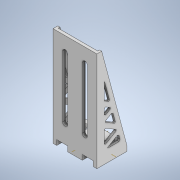
# Autodesk Inventor part: Bottom
Saved by Autodesk Inventor 2020 (Build 240168000, 168)
## iProperties
Created: 2019-08-01
Part Number: Bottom
Material: Generic
Document SubType Name: Modeling
Designer: Alex
Density: 1 g/cm^3
Appearance: Default
Author: Alex
Autodesk Inventor part; units mm, degrees
ref_plane "YZ Plane" through (0, 0, 0) normal (1, 0, 0) x (0, 1, 0)
ref_plane "XZ Plane" through (0, 0, 0) normal (0, 1, 0) x (-1, 0, 0)
ref_plane "XY Plane" through (0, 0, 0) normal (0, 0, 1) x (1, 0, 0)
sketch "Sketch1" plane through (0, 0, 0) normal (0, 1, 0) x (-1, 0, 0)
  line L0 (30, -20) -> (-30, -20)
  line L1 (-30, -20) -> (-30, 20)
  line L2 (-30, 20) -> (30, 20)
  line L3 (30, 20) -> (30, -20)
  line L4 (17.5, -11) -> (17.5, 5) construction
  line L5 (22, -11) -> (22, 5)
  line L6 (13, 5) -> (13, -11)
  arc A0 (13, -11) -> (22, -11) centre (17.5, -11) ccw
  arc A1 (22, 5) -> (13, 5) centre (17.5, 5) ccw
  line L7 (-17.5, -11) -> (-17.5, 5) construction
  line L8 (-13, -11) -> (-13, 5)
  line L9 (-22, 5) -> (-22, -11)
  arc A2 (-22, -11) -> (-13, -11) centre (-17.5, -11) ccw
  arc A3 (-13, 5) -> (-22, 5) centre (-17.5, 5) ccw
  line L10 (0, -28) -> (0, 28) construction
  line L11 (42, 0) -> (-42, 0) construction
  point P0 (0, 0)
  point P1 (17.5, -3)
  point P2 (-17.5, -3)
  dimension "d0" = 60
  dimension "d1" = 40
  dimension "d2" = 4.5
  dimension "d3" = 9
  dimension "d4" = 15
  dimension "d5" = 35
  constraints: 24 end point, 8 point on circle, 8 tangent, 6 parallel, 4 centre point, 2 midpoint, 1 equal radius, 1 horizontal, 1 horizontal alignment, 1 perpendicular, 1 vertical, 3 other
  measures "d0" distance of L1.end L2.end
  measures "d1" distance of L0.end L1.end
  measures "d2" radius of A0
  measures "d3" distance from line of L0 L4.start
  measures "d4" distance from line of L4.end L2
  measures "d5" distance of point (-17.5, -3) point (17.5, -3)
extrude "Extrusion1" add sketch "Sketch1" along normal blind 4
sketch "Sketch2" plane through (0, 4, 0) normal (0, 1, 0) x (1, 0, 0)
  line L0 (-30, -20) -> (30, -20) construction
  line L1 (30, -20) -> (30, 20) construction
  line L2 (30, 20) -> (-30, 20) construction
  line L3 (-30, 20) -> (-30, -20) construction
  line L4 (13, -5) -> (13, 11) construction
  arc A0 (22, 11) -> (13, 11) centre (17.5, 11) ccw construction
  line L5 (22, 11) -> (22, -5) construction
  arc A1 (13, -5) -> (22, -5) centre (17.5, -5) ccw construction
  arc A2 (-22, -5) -> (-13, -5) centre (-17.5, -5) ccw construction
  line L6 (-22, -5) -> (-22, 11) construction
  arc A3 (-13, 11) -> (-22, 11) centre (-17.5, 11) ccw construction
  line L7 (-13, 11) -> (-13, -5) construction
  line L8 (30, -20) -> (30, 20) construction
  line L9 (30, -20) -> (30, 20)
  line L10 (30, 20) -> (-30, 20) construction
  line L11 (27, 20) -> (27, -16)
  line L12 (27, -16) -> (-27, -16)
  line L13 (-27, -16) -> (-27, 20)
  line L14 (-30, 20) -> (-30, -20)
  line L15 (-30, -20) -> (30, -20) projected
  line L16 (-30, -20) -> (30, -20)
  line L17 (30, 20) -> (27, 20)
  line L18 (-27, 20) -> (-30, 20)
  line L19 (0, 38.5) -> (0, -38.5) construction
  point P0 (0, 0)
  dimension "d9" = 4
  dimension "d10" = 3
  constraints: 16 end point, 3 collinear, 3 perpendicular, 2 point on line, 1 vertical, 1 other
  measures "d9" distance between parallel lines of L0 L12
  measures "d10" distance between parallel lines of L11 L1
extrude "Extrusion2" add sketch "Sketch2" along normal blind 125
draft "FaceDraft1" angle 15 pull direction (0, 1, 0) fixed plane through (-4.3333, 4, -0.3333) normal (0, 1, 0) faces at (29, 44.3333, -20)
sketch "Sketch3" plane through (-30, 0, 20) normal (0, 0, 1) x (1, 0, 0)
  line L0 (0, 0) -> (60, 0) construction
  line L1 (60, 0) -> (60, 129) construction
  line L2 (0, 129) -> (60, 129) construction
  line L3 (0, 0) -> (0, 129) construction
  line L4 (16.5, 109) -> (16.5, 25) construction
  line L5 (13, 109) -> (13, 25)
  line L6 (20, 25) -> (20, 109)
  arc A0 (20, 109) -> (13, 109) centre (16.5, 109) ccw
  arc A1 (13, 25) -> (20, 25) centre (16.5, 25) ccw
  line L7 (43.5, 109) -> (43.5, 25) construction
  line L8 (40, 109) -> (40, 25)
  line L9 (47, 25) -> (47, 109)
  arc A2 (47, 109) -> (40, 109) centre (43.5, 109) ccw
  arc A3 (40, 25) -> (47, 25) centre (43.5, 25) ccw
  line L10 (0, 129) -> (60, 129) construction
  line L11 (30, 129) -> (30, 0) construction
  point P0 (16.5, 67)
  point P1 (43.5, 67)
  dimension "d17" = 3.5
  dimension "d18" = 20
  dimension "d19" = 25
  dimension "d20" = 10
  constraints: 18 end point, 8 point on circle, 8 tangent, 4 centre point, 4 parallel, 3 midpoint, 2 vertical, 1 equal radius, 1 horizontal alignment, 1 other
  measures "d17" radius of A0
  measures "d18" distance from line of L2 L4.start
  measures "d19" distance from line of L0 L4.end
  measures "d20" distance between parallel lines of L11 L8
extrude "Extrusion3" cut sketch "Sketch3" against normal up to next
sketch "Sketch5" plane through (0, 0, 0) normal (0, -1, 0) x (1, 0, 0)
  line L0 (30, -21.0718) -> (-30, -21.0718) construction
  line L1 (30, 20) -> (30, -21.0718) construction
  line L2 (-30, 20) -> (30, 20) construction
  line L3 (-30, -21.0718) -> (-30, 20) construction
  arc A0 (22, 5) -> (13, 5) centre (17.5, 5) ccw construction
  line L4 (22, -11) -> (22, 5) construction
  arc A1 (13, -11) -> (22, -11) centre (17.5, -11) ccw construction
  line L5 (13, 5) -> (13, -11) construction
  arc A2 (-22, -11) -> (-13, -11) centre (-17.5, -11) ccw construction
  line L6 (-22, 5) -> (-22, -11) construction
  arc A3 (-13, 5) -> (-22, 5) centre (-17.5, 5) ccw construction
  line L7 (-13, -11) -> (-13, 5) construction
  line L8 (30, -21.0718) -> (30, 20) projected
  line L9 (30, 20) -> (30, -21.0718)
  line L10 (25, 20) -> (25, -21.0718)
  line L11 (10, 20) -> (10, -21.0718)
  line L12 (17.5, 5) -> (17.5, -11) construction
  line L13 (-10, 20) -> (-10, -21.0718)
  line L14 (30, -21.0718) -> (-30, -21.0718) construction
  line L15 (-25, -21.0718) -> (-25, 20)
  line L16 (-30, 20) -> (30, 20) construction
  line L17 (0, -40.2471) -> (0, 38.7912) construction
  line L18 (25, 20) -> (30, 20)
  line L19 (10, 20) -> (-10, 20)
  line L20 (-25, 20) -> (-30, 20)
  line L21 (-30, -21.0718) -> (-30, 20) projected
  line L22 (-30, 20) -> (-30, -21.0718)
  line L23 (-30, -21.0718) -> (-25, -21.0718)
  line L24 (10, -21.0718) -> (-10, -21.0718)
  line L25 (25, -21.0718) -> (30, -21.0718)
  point P0 (0, 0)
  point P1 (30, 13.4936)
  point P2 (30, 14.4677)
  dimension "d27" = 15
  constraints: 26 end point, 8 point on line, 6 collinear, 4 perpendicular, 3 vertical, 3 other
  measures "d27" distance between parallel lines of L10 L11
extrude "Extrusion5" add sketch "Sketch5" along normal blind 7
sketch "Sketch6" plane through (-30, 129, 13.4936) normal (-1, 0, 0) x (0, 0, 1)
  line L0 (6.5064, -136) -> (6.5064, 0) construction
  line L1 (-34.5654, -129) -> (0, 0) construction
  line L2 (-34.5654, -129) -> (-34.5654, -136) construction
  line L3 (6.5064, -136) -> (-34.5654, -136) construction
  line L4 (-33.4936, -125) -> (2.5064, -125) construction
  line L5 (-33.4936, -125) -> (0, 0) construction
  line L6 (2.5064, 0) -> (0, 0) construction
  line L7 (-3.4936, -119) -> (-25.6743, -119) construction
  line L8 (-25.6743, -119) -> (-3.4936, -36.2207) construction
  line L9 (-3.4936, -36.2207) -> (-3.4936, -119) construction
  line L10 (-6.4936, -119) -> (-23.1046, -109.4097) construction
  line L11 (-21.4969, -103.4097) -> (-3.4936, -113.8038) construction
  line L12 (-21.4969, -103.4097) -> (-3.4936, -93.0155) construction
  line L13 (-19.3007, -95.2135) -> (-3.4936, -86.0873) construction
  line L14 (-15.0652, -79.4064) -> (-3.4936, -86.0873) construction
  line L15 (-13.4575, -73.4064) -> (-3.4936, -79.1591) construction
  line L16 (-11.2614, -65.2103) -> (-3.4936, -60.7256) construction
  line L17 (-13.4575, -73.4064) -> (-3.4936, -67.6538) construction
  line L18 (-3.4936, -113.8038) -> (-6.4936, -119) construction
  line L19 (-23.6743, -119) -> (-8.4936, -119)
  line L20 (-23.6222, -111.3415) -> (-25.1567, -117.0681)
  line L21 (-21.3725, -110.4097) -> (-8.2257, -118)
  line L22 (-17.5687, -94.2135) -> (-5.2257, -87.0873)
  line L23 (-13.3332, -80.4064) -> (-5.2257, -85.0873)
  line L24 (-15.5829, -81.3383) -> (-18.7831, -93.2817)
  line L25 (-11.7255, -74.4064) -> (-5.2257, -78.1591)
  line L26 (-3.4936, -69.6538) -> (-3.4936, -77.1591)
  line L27 (-11.7255, -72.4064) -> (-5.2257, -68.6538)
  line L28 (-9.5293, -64.2103) -> (-3.4936, -60.7256)
  line L29 (-3.4936, -38.2207) -> (-3.4936, -60.7256)
  line L30 (-10.7437, -63.2784) -> (-4.0113, -38.1525)
  line L31 (-19.7648, -104.4097) -> (-5.2257, -112.8038)
  line L32 (-3.4936, -95.0155) -> (-3.4936, -111.8038)
  line L33 (-19.7648, -102.4097) -> (-5.2257, -94.0155)
  line L34 (-25.1567, -117.0681) -> (-23.6743, -119)
  line L35 (-25.1567, -117.0681) -> (-23.6743, -119)
  line L36 (-8.2257, -118) -> (-8.4936, -119)
  line L37 (-23.6222, -111.3415) -> (-21.3725, -110.4097)
  line L38 (-5.2257, -112.8038) -> (-3.4936, -111.8038)
  line L39 (-5.2257, -112.8038) -> (-3.4936, -111.8038)
  line L40 (-5.2257, -94.0155) -> (-3.4936, -95.0155)
  line L41 (-19.7648, -102.4097) -> (-19.7648, -104.4097)
  line L42 (-17.5687, -94.2135) -> (-18.7831, -93.2817)
  line L43 (-5.2257, -87.0873) -> (-5.2257, -85.0873)
  line L44 (-13.3332, -80.4064) -> (-15.5829, -81.3383)
  line L45 (-5.2257, -68.6538) -> (-3.4936, -69.6538)
  line L46 (-5.2257, -78.1591) -> (-3.4936, -77.1591)
  line L47 (-11.7255, -74.4064) -> (-11.7255, -72.4064)
  line L48 (-9.5293, -64.2103) -> (-10.7437, -63.2784)
  line L49 (-9.5293, -64.2103) -> (-10.7437, -63.2784)
  line L50 (-4.0113, -38.1525) -> (-3.4936, -38.2207)
  line L51 (2.5064, -125) -> (2.5064, 0) projected
  line L52 (0, 0) -> (6.5064, 0) projected
  point P0 (-25.6743, -119)
  point P1 (-3.4936, -113.8038)
  dimension "d41" = 6
  dimension "d42" = 6
  dimension "d43" = 6
  dimension "d44" = 6
  dimension "d45" = 30
  dimension "d46" = 60
  dimension "d47" = 60
  dimension "d49" = 6
  dimension "d50" = 60
  dimension "d56" = 2
  dimension "d57" = 2
  dimension "d58" = 2
  dimension "d59" = 2
  dimension "d60" = 2
  dimension "d61" = 2
  dimension "d62" = 2
  dimension "d63" = 2
  dimension "d64" = 2
  dimension "d65" = 2
  dimension "d66" = 2
  dimension "d67" = 2
  dimension "d68" = 2
  dimension "d69" = 2
  dimension "d70" = 2
  dimension "d71" = 2
  dimension "d72" = 2
  dimension "d73" = 2
  dimension "d74" = 2
  dimension "d75" = 2
  dimension "d76" = 2
  dimension "d77" = 2
  dimension "d78" = 2
  dimension "d79" = 2
  dimension "d80" = 2
  dimension "d81" = 2
  dimension "d82" = 2
  dimension "d83" = 2
  dimension "d84" = 2
  dimension "d85" = 2
  dimension "d86" = 2
  dimension "d87" = 2
  dimension "d88" = 2
  dimension "d89" = 2
  dimension "d90" = 6
  constraints: 86 end point, 47 point on line, 10 collinear, 5 parallel, 1 perpendicular, 12 other
  measures "d41" distance between parallel lines of L4 L7
  measures "d42" distance between parallel lines of L11 L10
  measures "d43" distance between parallel lines of L13 L12
  measures "d44" distance between parallel lines of L15 L14
  measures "d45" angle of L7 L10
  measures "d46" angle of L12 L11
  measures "d47" angle of L14 L13
  measures "d49" distance between parallel lines of L16 L17
  measures "d50" angle of L15 L17
  measures "d56" distance of L34.start L7.end
  measures "d57" distance of L34.end L7.end
  measures "d58" distance of L20.end point (-25.674, -119)
  measures "d59" distance of L19.start point (-25.674, -119)
  measures "d60" distance of L21.end L10.start
  measures "d61" distance of L19.end L10.start
  measures "d62" distance of L20.start L10.end
  measures "d63" distance of L21.start L10.end
  measures "d64" distance of L38.start L11.end
  measures "d65" distance of L38.end L11.end
  measures "d66" distance of L31.end point (-3.494, -113.804)
  measures "d67" distance of L32.end point (-3.494, -113.804)
  measures "d68" distance of L33.end L12.end
  measures "d69" distance of L32.start L12.end
  measures "d70" distance of L33.start L11.start
  measures "d71" distance of L31.start L11.start
  measures "d72" distance of L22.start L13.start
  measures "d73" distance of L24.end L13.start
  measures "d74" distance of L22.end L13.end
  measures "d75" distance of L23.end L13.end
  measures "d76" distance of L23.start L14.start
  measures "d77" distance of L24.start L14.start
  measures "d78" distance of L27.end L17.end
  measures "d79" distance of L26.start L17.end
  measures "d80" distance of L25.end L15.end
  measures "d81" distance of L26.end L15.end
  measures "d82" distance of L25.start L15.start
  measures "d83" distance of L27.start L15.start
  measures "d84" distance of L48.start point (-11.261, -65.21)
  measures "d85" distance of L48.end point (-11.261, -65.21)
  measures "d86" distance of L28.start point (-11.261, -65.21)
  measures "d87" distance of L30.start point (-11.261, -65.21)
  measures "d88" distance of L30.end L9.start
  measures "d89" distance of L29.start L9.start
  measures "d90" distance between parallel lines of L51 L9
extrude "Extrusion7" cut sketch "Sketch6" against normal through all
sketch "Sketch4" plane through (-30, 0, 20) normal (0, 0, 1) x (1, 0, 0)
  arc A0 (40, 25) -> (47, 25) centre (38.5, 25) ccw construction
  line L0 (35, 25) -> (35, 109) construction
  arc A1 (47, 109) -> (40, 109) centre (38.5, 74) ccw construction
  line L1 (42, 109) -> (42, 25) construction
  line L2 (8, 25) -> (8, 74) construction
  arc A2 (15, 74) -> (8, 74) centre (11.5, 74) ccw construction
  line L3 (15, 74) -> (15, 25) construction
  arc A3 (8, 25) -> (15, 25) centre (11.5, 25) ccw construction
  line L4 (0, 0) -> (50, 0) construction
  line L5 (50, 0) -> (50, 94) construction
  line L6 (0, 94) -> (50, 94) construction
  line L7 (0, 0) -> (0, 94) construction
  line L8 (25, 62) -> (25, 37) construction
  line L9 (21, 62) -> (21, 37)
  line L10 (29, 37) -> (29, 62)
  arc A4 (29, 62) -> (21, 62) centre (25, 62) ccw
  arc A5 (21, 37) -> (29, 37) centre (25, 37) ccw
  arc A6 (40, 25) -> (47, 25) centre (43.5, 25) ccw construction
  line L11 (11.5, 74) -> (39.6645, 22.8866) construction
  arc A7 (47, 109) -> (40, 109) centre (43.5, 109) ccw construction
  line L12 (54.4585, 102.9617) -> (11.5, 25) construction
  point P0 (30, 0)
  point P1 (25, 49.5)
  dimension "d23" = 4
  dimension "d24" = 25
  constraints: 8 end point, 4 point on circle, 4 tangent, 2 centre point, 2 parallel, 1 midpoint, 10 other
  measures "d23" radius of A4
  measures "d24" distance of L8.end L8.start
equation "\"d42\" = d41"
equation "\"d43\" = d42"
equation "\"d44\" = d42"
equation "\"d49\" = d44"
body "Solid1"
